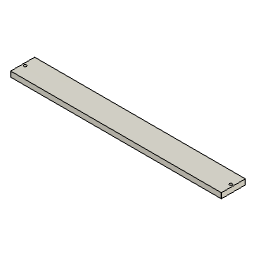
Chin Plate (Autodesk Fusion 360 design; units mm, degrees)
Autodesk Fusion 360 part; units mm, degrees
sketch "Sketch1" plane through (0, 0, 0) normal (0, 0, 1) x (1, 0, 0)
  line L0 (90, -10.25) -> (-90, -10.25)
  line L1 (-90, -10.25) -> (-90, 10.25)
  line L2 (-90, 10.25) -> (90, 10.25)
  line L3 (90, 10.25) -> (90, -10.25)
  line L4 (90, -10.25) -> (-90, 10.25) construction
  line L5 (-90, -10.25) -> (90, 10.25) construction
  line L6 (-87.75, 10.25) -> (-87.75, -10.25) construction
  line L7 (87.75, 10.25) -> (87.75, -10.25) construction
  circle A0 centre (-87.75, 0) radius 1.15
  circle A1 centre (87.75, 0) radius 1.15
  dimension "d1" = 180
  dimension "d2" = 20.5
  dimension "d3" = 2.25
  dimension "d4" = 2.25
  dimension "d5" = 2.3
  dimension "d6" = 2.3
  constraint horizontal L0
  constraint perpendicular L0 L1
  constraint parallel L0 L2
  constraint parallel L1 L3
  constraint coincident L4 origin
  constraint coincident L5 origin
  constraint coincident L2 L6.start
  constraint coincident L0 L6.end
  constraint perpendicular L0 L6
  constraint coincident L2 L7.start
  constraint coincident L0 L7.end
  constraint perpendicular L0 L7
  constraint midpoint L6 A0.centre
  constraint midpoint L7 A1.centre
  measures "d1" distance of L1.end L2.end
  measures "d2" distance of L0.end L1.end
  measures "d3" distance of L3 L7
  measures "d4" distance of L1 L6
  measures "d5" diameter of A0
  measures "d6" diameter of A1
extrude "Extrude1" add sketch "Sketch1" along normal blind 4.5
fillet "Fillet1" radius 0.1 4 edges at (90, -10.25, 2.25) (90, 10.25, 2.25) (-90, -10.25, 2.25) (-90, 10.25, 2.25)
